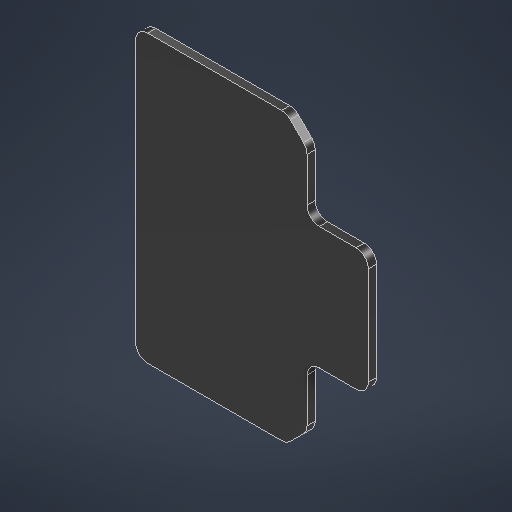
# Autodesk Inventor part: Second Layer Board
Saved by Autodesk Inventor 2026.1 (Build 301233020, 233B)
## iProperties
Created: 2026-04-04
Part Number: Second Layer Board
Material: Generic
Document SubType Name: Modeling
Designer: Bahaa
Density: 1 g/cm^3
Appearance: Glossy - Black
Mass: 6.72073 g
Surface Area: 72.0053 cm^2
Volume: 6.72073 cm^3
Author: Bahaa
Mass: 6.82073 g
Surface Area: 73.2053 cm^2
Volume: 6.82073 cm^3
Autodesk Inventor part; units mm, degrees
ref_plane "YZ Plane" through (0, 0, 0) normal (1, 0, 0) x (0, 1, 0)
ref_plane "XZ Plane" through (0, 0, 0) normal (0, 1, 0) x (-1, 0, 0)
ref_plane "XY Plane" through (0, 0, 0) normal (0, 0, 1) x (1, 0, 0)
sketch "Sketch1" plane through (0, 0, 0) normal (0, 1, 0) x (-1, 0, 0)
  line L0 (-16, 35) -> (21, 35)
  line L1 (21, 35) -> (21, -35)
  line L2 (21, -35) -> (-16, -35)
  line L3 (-21, -30) -> (-21, 30)
  line L4 (-21, 35) -> (21, -35) construction
  line L5 (21, 35) -> (-21, -35) construction
  line L6 (-36, -15) -> (-6, -15)
  line L7 (-6, -15) -> (-6, 15)
  line L8 (-6, 15) -> (-36, 15)
  line L9 (-36, 15) -> (-36, -15)
  line L10 (-36, -15) -> (-6, 15) construction
  line L11 (-6, -15) -> (-36, 15) construction
  line L12 (-16, -35) -> (-21, -30)
  line L13 (-21, 30) -> (-16, 35)
  point P0 (0, 0)
  point P1 (-21, 0)
  point P2 (-21, -15)
  point P3 (-21, 15)
  dimension "d0" = 42
  dimension "d1" = 70
  dimension "d10" = 30
  dimension "d11" = 30
  dimension "d12" = 5
  dimension "d13" = 5
  dimension "d14" = 5
  dimension "d15" = 5
  constraints: 28 end point, 5 midpoint, 4 parallel, 4 point on line, 2 horizontal, 2 perpendicular
  measures "d0" distance of L1.end L5.end
  measures "d1" distance of L0.end L1.end
  measures "d10" distance of L8.end L7.end
  measures "d11" distance of L7.end L6.end
  measures "d12" distance of L2.end L5.end
  measures "d13" distance of L3.start L5.end
  measures "d14" distance of L3.end L4.start
  measures "d15" distance of L0.start L4.start
extrude "Extrusion1" add sketch "Sketch1" along normal blind 2
fillet "Fillet1" radius 3 10 edges at (36, 1, -15) (36, 1, 15) (21, 1, -30) (16, 1, -35) (21, 1, 30) (16, 1, 35) (-21, 1, 35) (-21, 1, -35) (21, 1, -15) (21, 1, 15)
equation "\"d13\" = d12"
equation "\"d14\" = d12"
equation "\"d15\" = d14"
body "Solid1"
